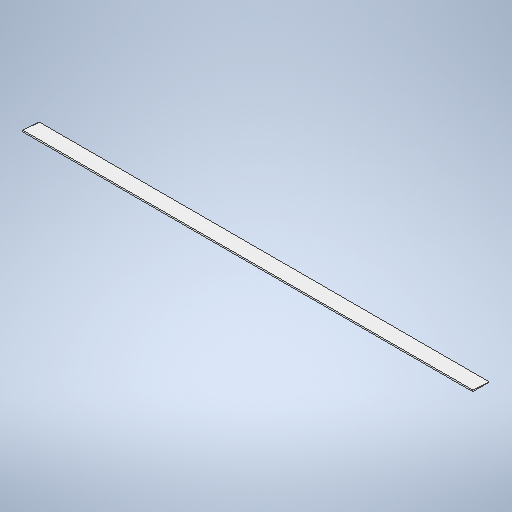
# Autodesk Inventor part: Intake_Vent
Saved by Autodesk Inventor 2025.1 (Build 291241020, 241B)
## iProperties
Created: 2024-10-02
Part Number: Intake_Vent
Material: Polystyrene
Document SubType Name: Modeling
Designer: Tom
Density: 1.021 g/cm^3
Appearance: Smooth - White
Author: Tom
Autodesk Inventor part; units mm, degrees
ref_plane "YZ Plane" through (0, 0, 0) normal (1, 0, 0) x (0, 1, 0)
ref_plane "XZ Plane" through (0, 0, 0) normal (0, 1, 0) x (-1, 0, 0)
ref_plane "XY Plane" through (0, 0, 0) normal (0, 0, 1) x (1, 0, 0)
sketch "Sketch1" plane through (0, 0, 0) normal (1, 0, 0) x (0, 1, 0)
  line L0 (0, 0) -> (25.4, 0)
  line L1 (25.4, 0) -> (0, -279.4)
  line L2 (0, -279.4) -> (0, 0)
  dimension "d0" = 279.4
  dimension "d1" = 25.4
  constraints: 6 end point, 1 horizontal, 1 perpendicular
  measures "d0" distance of L1.end L0.start
  measures "d1" distance of L0.start L0.end
extrude "Extrusion1" add sketch "Sketch1" along normal blind 7488.555
body "Solid1"
